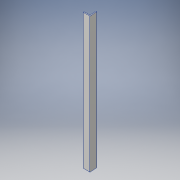
# Autodesk Inventor part: AngleL
Saved by Autodesk Inventor 2016 (Build 200138000, 138)
## iProperties
Created: 2018-05-16
Part Number: AngleL
Material: Aluminum 6061
Document SubType Name: Modeling
Designer: Kade
Density: 2.7 g/cm^3
Appearance: Aluminum - Flat
Mass: 375.703 g
Surface Area: 937.99 cm^2
Volume: 139.149 cm^3
Author: Kade
Autodesk Inventor part; units mm, degrees
ref_plane "YZ Plane" through (0, 0, 0) normal (1, 0, 0) x (0, 1, 0)
ref_plane "XZ Plane" through (0, 0, 0) normal (0, 1, 0) x (-1, 0, 0)
ref_plane "XY Plane" through (0, 0, 0) normal (0, 0, 1) x (1, 0, 0)
sketch "Sketch1" plane through (0, 0, 0) normal (0, 1, 0) x (-1, 0, 0)
  line L0 (0, 0) -> (25.4, 0)
  line L1 (25.4, 0) -> (25.4, -3.175)
  line L2 (25.4, -3.175) -> (3.175, -3.175)
  line L3 (3.175, -3.175) -> (3.175, -25.4)
  line L4 (3.175, -25.4) -> (0, -25.4)
  line L5 (0, -25.4) -> (0, 0)
  dimension "d0" = 25.4
  dimension "d1" = 3.175
  dimension "d2" = 90
  dimension "d7" = 25.4
  dimension "d8" = 3.175
  constraints: 12 end point, 2 horizontal, 2 perpendicular, 1 vertical
  measures "d0" distance of L0.start L0.end
  measures "d1" distance of L0.end L1.end
  measures "d2" angle of L0 L1
  measures "d7" distance of L4.end L0.start
  measures "d8" distance of L3.end L4.end
extrude "Extrusion1" add sketch "Sketch1" along normal blind 511.8354
sketch "Sketch2" plane through (0, 0, 0) normal (1, 0, 0) x (0, 0, -1)
  line L0 (25.4, 0) -> (25.4, 511.8354) projected
  line L1 (25.4, 511.8354) -> (50.8817, 511.8354) construction
  line L2 (0, 511.8354) -> (25.4, 511.8354) projected
  line L3 (25.4, 511.8354) -> (0, 509.7962)
  line L4 (0, 0) -> (0, 511.8354) projected
  line L5 (25.4, 511.8354) -> (50.8817, 511.8354) construction
  line L6 (0, 509.7962) -> (0, 511.8354)
  line L7 (25.4, 511.8354) -> (0, 511.8354)
  line L8 (25.4, 0) -> (0, 0) projected
  line L9 (0, 0) -> (25.4, 2.0392)
  line L10 (0, 0) -> (25.4817, 0) construction
  line L11 (25.4, 2.0392) -> (25.4, 0)
  line L12 (25.4, 0) -> (0, 0)
  dimension "d10" = 175.41
  dimension "d11" = 4.59
  constraints: 18 end point, 3 collinear, 3 horizontal, 2 equal length, 2 point on line
  measures "d10" angle of L3 L5
  measures "d11" angle of L10 L9
extrude "Extrusion2" cut sketch "Sketch2" against normal through all contours L8 L9 L0 | L3 L4 L2
body "Solid1"
